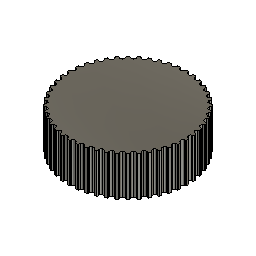
gear_48z (Autodesk Fusion 360 design; units mm, degrees)
Autodesk Fusion 360 part; units mm, degrees
sketch "Sketch1" plane through (0, 0, 0) normal (0, 0, 1) x (1, 0, 0) in component "gt2 pulley"
  circle A0 centre (0, 0) radius 15.2789 construction
  circle A1 centre (0, 0) radius 14.2749 construction
  line L0 (0, 0) -> (0, 15.2789) construction
  line L1 (0, 0) -> (0.9993, 15.2462) construction
  line L2 (0, 0) -> (1.4074, 15.2139) construction
  circle A2 centre (0, 0) radius 15.0249 construction
  arc A3 (0.387, 14.8845) -> (0.4534, 14.595) centre (1.384, 14.961) ccw
  circle A4 centre (0, 0) radius 14.8749 construction
  arc A5 (0.2397, 15.023) -> (0, 15.0249) centre (0, 0) ccw
  arc A6 (0.387, 14.8845) -> (0.2397, 15.023) centre (0.2374, 14.873) ccw
  arc A7 (0.4534, 14.595) -> (0.9336, 14.2443) centre (0.9699, 14.7981) ccw
  arc A8 (0, 15.0249) -> (-0.2397, 15.023) centre (0, 0) ccw
  arc A9 (-0.2397, 15.023) -> (-0.387, 14.8845) centre (-0.2374, 14.873) ccw
  arc A10 (-0.4534, 14.595) -> (-0.387, 14.8845) centre (-1.384, 14.961) ccw
  arc A11 (-0.9336, 14.2443) -> (-0.4534, 14.595) centre (-0.9699, 14.7981) ccw
  arc A12 (0.9336, 14.2443) -> (-0.9336, 14.2443) centre (0, 0) ccw
  point P0 (1.384, 14.961)
  point P1 (0, 15.0249)
  dimension "d18" = 30.5577
  dimension "d19" = 3.75
  dimension "d22" = 1.004
  dimension "d24" = 0.75
  dimension "d26" = 1
  dimension "d27" = 0.15
  dimension "d28" = 0.15
  dimension "d47" = 0.555
  dimension "d52" = 3.812
  constraint coincident A0.centre A1.centre
  constraint coincident A0 L0.end
  constraint vertical L0
  constraint coincident A0 L1.end
  constraint coincident A0 L2.end
  constraint concentric A1 A2
  constraint coincident A1 A7.end
  constraint coincident L1 A7.end
  constraint coincident A2 P0
  constraint coincident L2 P0
  constraint coincident P0 A3.centre
  constraint coincident A2 P1
  constraint coincident L0 P1
  constraint concentric A2 A4
  constraint coincident P1 A5.end
  constraint coincident A4 A6.centre
  constraint coincident A3.start A6.start
  constraint tangent A3 A6
  constraint tangent A3 A7
  constraint symmetric L0 A7.end A11.start
  constraint symmetric L0 A3.start A9.end
  constraint symmetric L0 A3.end A10.start
  constraint symmetric L0 A3 A10
  constraint symmetric L0 A5.start A8.end
  constraint symmetric L0 P1 A5.end
  constraint symmetric L0 A5 A8
  constraint symmetric L0 A6 A9
  constraint symmetric L0 A7 A11
  constraint coincident A1 A11.start
  constraint tangent A1 A7
  constraint coincident L1 A7.centre
  measures "d18" diameter of A0
  measures "d19" angle of L0 L1
  measures "d22" distance of A0 A1
  measures "d24" distance of A1 A2
  measures "d26" radius of A3
  measures "d27" distance of A2 A4
  measures "d28" radius of A6
  measures "d47" radius of A7
extrude "Extrude1" add sketch "Sketch1" along normal blind 10 makes body 1
pattern_circular "C-Pattern1" count 48 over 360 about axis through (0, 0, 1.75) along (0, 0, 1) of bodies 1 makes body 2 at (-2.581, 14.0396, 6.6667) makes body 3 at (-4.3914, 13.5826, 6.6667) makes body 4 at (-5.5585, 13.1482, 6.6667) makes body 5 at (-6.4991, 12.7096, 3.3333) makes body 6 at (-8.7721, 11.2615, 6.6667) makes body 7 at (-9.5672, 10.5944, 3.3333) makes body 8 at (-11.7525, 8.1025, 6.6667) makes body 9 at (-11.9832, 7.7572, 3.3333) makes body 10 at (-13.2276, 5.3667, 6.6667) makes body 11 at (-13.9586, 2.9882, 6.6667) makes body 12 at (-14.1659, 1.7603, 6.6667) makes body 13 at (-14.2564, -0.7264, 6.6667) makes body 14 at (-14.0396, -2.581, 6.6667) makes body 15 at (-13.7612, -3.7948, 6.6667) makes body 16 at (-12.8932, -6.1267, 6.6667) makes body 17 at (-12.3102, -7.2272, 6.6667) makes body 18 at (-11.2615, -8.7721, 6.6667) makes body 19 at (-10.5944, -9.5672, 3.3333) makes body 20 at (-8.1025, -11.7525, 6.6667) makes body 21 at (-7.0473, -12.414, 6.6667) makes body 22 at (-4.7846, -13.4491, 6.6667) makes body 23 at (-3.5942, -13.815, 6.6667) makes body 24 at (-1.1407, -14.2292, 6.6667) makes body 25 at (0.7264, -14.2564, 6.6667) makes body 26 at (2.581, -14.0396, 6.6667) makes body 27 at (3.7948, -13.7612, 6.6667) makes body 28 at (6.1267, -12.8932, 6.6667) makes body 29 at (7.2272, -12.3102, 6.6667) makes body 30 at (8.7721, -11.2615, 6.6667) makes body 31 at (9.5672, -10.5944, 3.3333) makes body 32 at (11.7525, -8.1025, 6.6667) makes body 33 at (11.9832, -7.7572, 3.3333) makes body 34 at (13.4491, -4.7846, 6.6667) makes body 35 at (13.9586, -2.9882, 6.6667) makes body 36 at (14.1659, -1.7603, 6.6667) makes body 37 at (14.2564, 0.7264, 6.6667) makes body 38 at (14.0396, 2.581, 6.6667) makes body 39 at (13.5826, 4.3914, 6.6667) makes body 40 at (12.8932, 6.1267, 6.6667) makes body 41 at (12.3102, 7.2272, 6.6667) makes body 42 at (10.8682, 9.255, 6.6667) makes body 43 at (10.5944, 9.5672, 3.3333) makes body 44 at (8.1025, 11.7525, 6.6667) makes body 45 at (7.7572, 11.9832, 3.3333) makes body 46 at (5.3667, 13.2276, 6.6667) makes body 47 at (4.3914, 13.5826, 3.3333) makes body 48 at (1.1407, 14.2292, 6.6667)
sketch "Sketch2" plane through (0, 0, 10) normal (0, 0, 1) x (-1, 0, 0)
  arc A0 (-9.3681, -11.5731) -> (-9.3356, -11.7726) centre (-9.2425, -11.655) ccw
  arc A1 (-9.3356, -11.7726) -> (-8.9552, -12.0645) centre (0, 0) ccw
  arc A2 (-8.9552, -12.0645) -> (-8.7541, -12.0442) centre (-8.8657, -11.9441) ccw
  arc A3 (-8.5251, -11.855) -> (-8.7541, -12.0442) centre (-8.0096, -12.7119) ccw
  arc A4 (-7.9307, -11.8691) -> (-8.5251, -11.855) centre (-8.239, -12.3306) ccw
  arc A5 (-9.4121, -10.7324) -> (-7.9307, -11.8691) centre (0, 0) ccw
  arc A6 (-9.2446, -11.303) -> (-9.4121, -10.7324) centre (-9.778, -11.1497) ccw
  arc A7 (-9.3681, -11.5731) -> (-9.2446, -11.303) centre (-10.2057, -11.0268) ccw
  circle A8 centre (0, 0) radius 14.2749
  constraint coincident A1.centre A5.centre
extrude "Extrude2" add sketch "Sketch2" against normal blind 10 contours A5 A8 bodies 1 2 3 4 5 6 7 8 9 10 11 12 13 14 15 16 17 18 19 20 21 22 23 24 25 26 27 28 29 30 31 32 33 34 35 36 37 38 39 40 41 42 43 44 45 46 47 48
extrude "Extrude4" [suppressed] in component "gt2 pulley"
pattern_circular "C-Pattern7" [suppressed] in component "gt2 pulley"
extrude "Extrude3" [suppressed] in component "gt2 pulley"
pattern_circular "C-Pattern6" [suppressed] in component "gt2 pulley"
extrude "Extrude2'" [suppressed] in component "gt2 pulley"
pattern_circular "C-Pattern5" [suppressed] in component "gt2 pulley"
extrude "Extrude1'" [suppressed] in component "gt2 pulley"
pattern_circular "C-Pattern4" [suppressed] in component "gt2 pulley"
pattern_circular "C-Pattern3" [suppressed] in component "gt2 pulley"
pattern_circular "C-Pattern2" [suppressed] in component "gt2 pulley"
pattern_circular "C-Pattern1'" [suppressed] in component "gt2 pulley"
copy_body "Body->Comp1" [suppressed] in component "Component"
copy_body "Body->Comp2" [suppressed] in component "Component'"
copy_body "Body->Comp3" [suppressed] in component "Component''"
copy_body "Body->Comp4" [suppressed] in component "Component'''"
copy_body "Body->Comp5" [suppressed] in component "Component''''"
copy_body "Body->Comp6" [suppressed] in component "Component'''''"
copy_body "Body->Comp7" [suppressed] in component "Component''''''"
copy_body "Body->Comp8" [suppressed] in component "Component'''''''"
copy_body "Body->Comp9" [suppressed] in component "Component''''''''"
copy_body "Body->Comp10" [suppressed] in component "Component'''''''''"
copy_body "Body->Comp11" [suppressed] in component "Component''''''''''"
copy_body "Body->Comp12" [suppressed] in component "Component'''''''''''"
copy_body "Body->Comp13" [suppressed] in component "Component''''''''''''"
copy_body "Body->Comp14" [suppressed] in component "Component'''''''''''''"
copy_body "Body->Comp15" [suppressed] in component "Component''''''''''''''"
copy_body "Body->Comp16" [suppressed] in component "Component'''''''''''''''"
copy_body "Body->Comp17" [suppressed] in component "Component''''''''''''''''"
copy_body "Body->Comp18" [suppressed] in component "Component'''''''''''''''''"
copy_body "Body->Comp19" [suppressed] in component "Component''''''''''''''''''"
copy_body "Body->Comp20" [suppressed] in component "Component'''''''''''''''''''"
component "gt2 pulley" placed x (1, 0, 0) y (0, 1, 0) z (0, 0, 1) at (0, 0, 0)
equation "NumTeeth = 48" comment "min 20"
equation "ToothPitch = 2 mm"
equation "PullyDia = NumTeeth * ToothPitch / PI"
equation "ToothAng = ( ( 360 / NumTeeth ) * 1 deg )"
equation "TransOffsetAngle = ToothAng * 0.2"
equation "Sholulder_Radius = 0.15 mm"
equation "Root_Radius = 0.555 mm"
equation "TransRadius = 1 mm"
equation "ToolHeight = 0.75 mm"
equation "PLD = 0.254 mm"
equation "d18 = PullyDia"
equation "d19 = ToothAng / 2"
equation "d22 = PLD + ToolHeight"
equation "d24 = ToolHeight"
equation "d26 = TransRadius"
equation "d27 = Sholulder_Radius"
equation "d31 = NumTeeth"
equation "d33 = NumTeeth"
equation "d35 = NumTeeth"
equation "d37 = NumTeeth"
equation "d41 = NumTeeth"
equation "d45 = NumTeeth"
equation "d47 = Root_Radius"
equation "d50 = NumTeeth"
